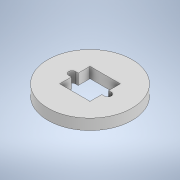
# Autodesk Inventor part: circle_cutout
Saved by Autodesk Inventor 2020 (Build 240168000, 168)
## iProperties
Created: 2024-03-15
Part Number: circle_cutout
Material: Типовые
Document SubType Name: Modeling
Designer: 4s
Density: 1 g/cm^3
Appearance: По умолчанию
Author: 4s
Autodesk Inventor part; units mm, degrees
ref_plane "YZ Plane" through (0, 0, 0) normal (1, 0, 0) x (0, 1, 0)
ref_plane "XZ Plane" through (0, 0, 0) normal (0, 1, 0) x (-1, 0, 0)
ref_plane "XY Plane" through (0, 0, 0) normal (0, 0, 1) x (1, 0, 0)
sketch "Эскиз1" plane through (0, 0, 0) normal (0, 1, 0) x (-1, 0, 0)
  line L0 (8.5, -8.5) -> (-8.5, -8.5)
  line L1 (-8.5, -8.5) -> (-8.5, -1.9)
  line L2 (-8.5, 8.5) -> (8.5, 8.5)
  line L3 (8.5, 8.5) -> (8.5, 1.9)
  line L4 (0, 0) -> (0, -10.3494) construction
  line L5 (0, 0) -> (-17.6402, 0) construction
  circle A0 centre (10, 0) radius 0.9 construction
  circle A1 centre (-10, 0) radius 0.9 construction
  arc A2 (10, -1.9) -> (10, 1.9) centre (10, 0) ccw
  line L6 (10, -1.9) -> (8.5, -1.9)
  line L7 (10, 1.9) -> (8.5, 1.9)
  line L8 (8.5, -1.9) -> (8.5, -8.5)
  line L9 (8.5, 1.9) -> (8.5, -1.9) construction
  circle A3 centre (-10, 0) radius 0.9 construction
  arc A4 (-10, 1.9) -> (-10, -1.9) centre (-10, 0) ccw
  line L10 (-10, -1.9) -> (-8.5, -1.9)
  line L11 (-10, 1.9) -> (-8.5, 1.9)
  line L12 (-8.5, -1.9) -> (-8.5, 1.9) construction
  line L13 (-8.5, 1.9) -> (-8.5, 8.5)
  circle A5 centre (0, 0) radius 23.5
  dimension "d0" = 17
  dimension "d1" = 17
  dimension "d2" = 1.8
  dimension "d3" = 20
  dimension "d4" = 3.8
  dimension "d5" = 47
  constraints: 28 end point, 11 parallel, 9 symmetric about line, 6 centre point, 4 point on circle, 3 coincident, 3 perpendicular, 2 horizontal, 1 point on line, 1 tangent, 1 vertical, 5 other
  measures "d0" distance between parallel lines of L1 L3
  measures "d1" distance between parallel lines of L2 L0
  measures "d2" diameter of A0
  measures "d3" distance of A1.centre A0.centre
  measures "d4" diameter of A2
  measures "d5" diameter of A5
extrude "Выдавливание1" add sketch "Эскиз1" along normal blind 6
